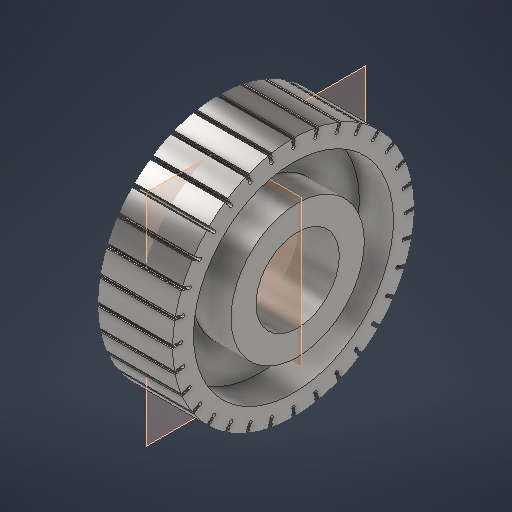
# Autodesk Inventor part: DiscoPaleSatdio3-DimensioniAprossimate
Saved by Autodesk Inventor 2026.2 (Build 302298010, 298A)
## iProperties
Created: 2026-04-19
Part Number: DiscoPaleSatdio3-DimensioniAprossimate
Material: Steel, Alloy
Document SubType Name: Modeling
Designer: Yan
Density: 7.73 g/cm^3
Appearance: Semi-Polished
Author: Yan
Autodesk Inventor part; units mm, degrees
ref_plane "XZ Plane" through (0, 0, 0) normal (0, 1, 0) x (-1, 0, 0)
sketch "Sketch1" plane through (0, 0, 0) normal (1, 0, 0) x (0, 1, 0)
  circle A0 centre (0, 0) radius 50
  circle A1 centre (0, 0) radius 80
  dimension "d0" = 100
  dimension "d1" = 160
  constraints: 2 centre point, 2 coincident
  measures "d0" diameter of A0
  measures "d1" diameter of A1
extrude "Extrusion1" add sketch "Sketch1" along normal blind 100
ref_plane "Work Plane1" through (0, 0, 0) normal (0, 0, 1) x (1, 0, 0)
sketch "Sketch2" plane through (0, 0, 0) normal (0, 0, 1) x (1, 0, 0)
  line L0 (0, 80) -> (100, 80) projected
  line L1 (54, 80) -> (54, 120)
  line L2 (54, 120) -> (46, 120)
  line L3 (46, 120) -> (46, 80)
  line L4 (0, -80) -> (0, 80) projected
  line L5 (-20, 0) -> (120, 0) projected
  point P0 (0, 0)
  dimension "d5" = 8
  dimension "d6" = 46
  dimension "d7" = 40
  constraints: 6 end point, 2 perpendicular, 2 point on line, 1 vertical
  measures "d5" distance between parallel lines of L3 L1
  measures "d6" distance between parallel lines of L4 L3
  measures "d7" distance between parallel lines of L0 L2
revolve "Revolution1" add sketch "Sketch2" angle 360 about axis through (-10, 0, 0) along (1, 0, 0)
ref_plane "Work Plane2" through (50, 0, 0) normal (1, 0, 0) x (0, 1, 0)
sketch "Sketch4" plane through (50, 0, 0) normal (1, 0, 0) x (0, 1, 0)
  circle A0 centre (0, 0) radius 145
  circle A1 centre (0, 0) radius 120
  dimension "d12" = 290
  dimension "d13" = 240
  constraints: 2 centre point, 2 coincident
  measures "d12" diameter of A0
  measures "d13" diameter of A1
extrude "Extrusion2" add sketch "Sketch4" along normal mid plane 90
sketch "Sketch5" plane through (95, 0, 0) normal (1, 0, 0) x (0, 0, -1)
  line L0 (-2.1774, 145) -> (-1.6, 144)
  line L1 (-1.6, 144) -> (-1.6, 143)
  circle A0 centre (0, 0) radius 145 projected
  line L2 (-1.6, 143) -> (-2, 142.3072)
  line L3 (-2, 142.3072) -> (-2, 141.3072)
  line L4 (-2, 141.3072) -> (-1.3, 140.0947)
  line L5 (-1.3, 140.0947) -> (-1.3, 139.0947)
  line L6 (-1.3, 139.0947) -> (-1.6, 138.5751)
  line L7 (-1.6, 138.5751) -> (-1.6, 137.5751)
  line L8 (-1.6, 137.5751) -> (-1.3, 137.0555)
  line L9 (-1.3, 137.0555) -> (-1.3, 136.5199)
  line L10 (0, 145) -> (0, 135)
  line L11 (2.1774, 145) -> (1.6, 144)
  line L12 (1.6, 144) -> (1.6, 143)
  line L13 (1.6, 143) -> (2, 142.3072)
  line L14 (2, 142.3072) -> (2, 141.3072)
  line L15 (2, 141.3072) -> (1.3, 140.0947)
  line L16 (1.3, 140.0947) -> (1.3, 139.0947)
  line L17 (1.3, 139.0947) -> (1.6, 138.5751)
  line L18 (1.6, 138.5751) -> (1.6, 137.5751)
  line L19 (1.6, 137.5751) -> (1.3, 137.0555)
  line L20 (1.3, 137.0555) -> (1.3, 136.5199)
  line L21 (-2.1774, 145) -> (2.1774, 145)
  arc A1 (-1.3, 136.5199) -> (1.3, 136.5199) centre (0, 135) ccw
  point P0 (2.168, 144.9838)
  point P1 (-2.168, 144.9838)
  point P2 (0, 145)
  point P3 (0, 133)
  dimension "d30" = 1.6
  dimension "d31" = 2
  dimension "d32" = 1.3
  dimension "d33" = 1.6
  dimension "d34" = 2
  dimension "d36" = 145
  dimension "d37" = 1
  dimension "d38" = 1
  dimension "d40" = 1
  dimension "d43" = 1
  dimension "d44" = 10
  dimension "d46" = 0
  dimension "d48" = 30
  dimension "d50" = 30
  dimension "d51" = 30
  dimension "d52" = 30
  dimension "d60" = 1
  dimension "d64" = 12
  constraints: 44 end point, 11 symmetric about line, 5 vertical, 3 point on circle, 2 parallel, 2 point on line, 1 centre point, 1 horizontal, 1 midpoint
  measures "d30" distance between parallel lines of L10 L1
  measures "d31" distance between parallel lines of L10 L3
  measures "d32" distance between parallel lines of L10 L5
  measures "d33" distance between parallel lines of L10 L7
  measures "d34" radius of A1
  measures "d36" distance from line of A0.centre L21
  measures "d37" vertical distance of L0.start L0.end
  measures "d38" distance of L0.end L1.end
  measures "d40" distance of L2.end L3.end
  measures "d43" distance of L6.end L7.end
  measures "d44" distance of L10.start L10.end
  measures "d46" distance from line of point (0, 0) L10
  measures "d48" angle of L10 L6
  measures "d50" angle of L10 L4
  measures "d51" angle of L10 L0
  measures "d52" angle of L10 L2
  measures "d60" distance of L4.end L5.end
  measures "d64" distance from line of L21 point (0, 133)
extrude "Extrusion3" cut sketch "Sketch5" against normal blind 90 contours A0 L11 L12 L13 L14 L15 L16 L17 L18 L19 L20 A1 L9 L8 L7 L6 L5 L4 L3 L2 L1 L0 picked at (-0.3119, 135.424)
pattern_circular "Circular Pattern1" count 32 over 360 about axis through (-10, 0, 0) along (1, 0, 0) of "Extrusion3"
body "Solid1"
